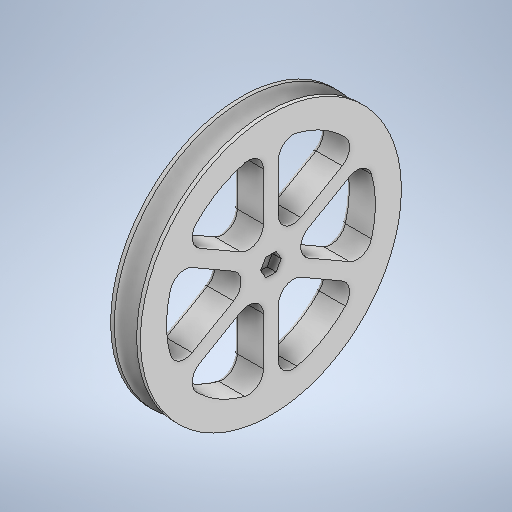
# Autodesk Inventor part: PLA Wheel Frame
Saved by Autodesk Inventor 2025.2 (Build 292293000, 293)
## iProperties
Created: 2025-01-16
Part Number: PLA Wheel Frame
Material: Generic
Document SubType Name: Modeling
Designer: Matt Tidd
Density: 1 g/cm^3
Appearance: Default
Author: Matt Tidd
Autodesk Inventor part; units mm, degrees
ref_plane "YZ Plane" through (0, 0, 0) normal (1, 0, 0) x (0, 1, 0)
ref_plane "XZ Plane" through (0, 0, 0) normal (0, 1, 0) x (-1, 0, 0)
ref_plane "XY Plane" through (0, 0, 0) normal (0, 0, 1) x (1, 0, 0)
sketch "Sketch1" plane through (0, 0, 0) normal (1, 0, 0) x (0, 1, 0)
  circle A0 centre (0, 0) radius 6
  line L0 (6, 3.4737) -> (6.0083, -3.4593)
  line L1 (6.0083, -3.4593) -> (0.0083, -6.933)
  line L2 (0.0083, -6.933) -> (-6, -3.4737)
  line L3 (-6, -3.4737) -> (-6.0083, 3.4593)
  line L4 (-6.0083, 3.4593) -> (-0.0083, 6.933)
  line L5 (-0.0083, 6.933) -> (6, 3.4737)
  circle A1 centre (0, 0) radius 20
  dimension "d0" = 12
  dimension "d1" = 40
  constraints: 12 end point, 3 coincident, 2 centre point, 13 other
  measures "d0" diameter of A0
  measures "d1" diameter of A1
extrude "Extrusion1" add sketch "Sketch1" along normal blind 20 contours A0 | L0 L1 L2 L3 L4 L5 | A1
sketch "Sketch2" plane through (20, 0, 0) normal (1, 0, 0) x (0, 0, -1)
  circle A0 centre (0, 0) radius 6
  line L0 (-6.934, 0) -> (-3.467, 6.005)
  line L1 (-3.467, 6.005) -> (3.467, 6.005)
  line L2 (3.467, 6.005) -> (6.934, 0)
  line L3 (6.934, 0) -> (3.467, -6.005)
  line L4 (3.467, -6.005) -> (-3.467, -6.005)
  line L5 (-3.467, -6.005) -> (-6.934, 0)
  point P0 (0, 6)
  dimension "d4" = 12
  constraints: 12 end point, 2 coincident, 1 vertical alignment, 15 other
extrude "Extrusion2" cut sketch "Sketch2" against normal blind 6 contours A0 | L0 L1 L2 L3 L4 L5
sketch "Sketch3" plane through (0, 0, 0) normal (-1, 0, 0) x (0, 0, 1)
  circle A0 centre (0, 0) radius 15
  dimension "d7" = 30
  constraints: 1 centre point, 1 coincident
  measures "d7" diameter of A0
extrude "Extrusion3" cut sketch "Sketch3" against normal blind 6
sketch "Sketch4" plane through (6, 0, 0) normal (-1, 0, 0) x (0, 0, 1)
  circle A0 centre (0, 0) radius 6
  dimension "d10" = 12
  constraints: 1 centre point, 1 coincident
  measures "d10" diameter of A0
extrude "Extrusion4" cut sketch "Sketch4" against normal blind 2
sketch "Sketch5" plane through (8, 0, 0) normal (-1, 0, 0) x (0, 0, 1)
  circle A0 centre (0, 0) radius 1.5
  dimension "d13" = 3
  constraints: 1 centre point, 1 coincident
  measures "d13" diameter of A0
extrude "Extrusion5" cut sketch "Sketch5" against normal through all
sketch "Sketch6" plane through (0, 0, 0) normal (-1, 0, 0) x (0, 0, 1)
  circle A0 centre (0, 0) radius 20 projected
  point P0 (0, 20)
  constraints: 1 vertical alignment, 1 other
ref_plane "Work Plane1" through (0, 20, 0) normal (0, 1, 0) x (-1, 0, 0)
sketch "Sketch7" plane through (0, 20, 0) normal (0, 1, 0) x (-1, 0, 0)
  line L0 (0, 0) -> (-20, 0) construction
  line L1 (-20, -3.467) -> (-20, 3.467) construction
  line L2 (-20, 5) -> (-20, -5) construction
  line L3 (-20, -3.467) -> (-20, -6.934) construction
  line L4 (-20, -5) -> (0, -5) construction
  line L5 (-20, -5) -> (0, -5)
  line L6 (0, -5) -> (0, 5)
  line L7 (0, 5) -> (-20, 5)
  line L8 (-20, 5) -> (-20, -5)
  dimension "d22" = 10
  dimension "d23" = 20
  dimension "d24" = 90
  dimension "d25" = 20
  dimension "d26" = 10
  constraints: 14 end point, 2 parallel, 2 perpendicular, 1 horizontal, 1 midpoint, 1 point on line
  measures "d22" distance of L2.start L2.end
  measures "d23" distance of L2.end L4.end
  measures "d24" angle of L4 L2
  measures "d25" distance of L7.end L6.end
  measures "d26" distance of L6.end L5.end
extrude "Extrusion6" add sketch "Sketch7" along normal blind 50 and the other way blind 2
pattern_circular "Circular Pattern1" count 6 over 360 about axis through (8, 0, 0) along (1, 0, 0) of "Extrusion6"
fillet "Fillet1" radius 10 12 edges at (10, 19.3649, 5) (10, 19.3649, -5) (10, 14.0126, -14.2705) (10, 5.3523, -19.2705) (10, -5.3523, -19.2705) (10, -14.0126, -14.2705) (10, -19.3649, -5) (10, -19.3649, 5) (10, -14.0126, 14.2705) (10, -5.3523, 19.2705) (10, 5.3523, 19.2705) (10, 14.0126, 14.2705)
sketch "Sketch9" plane through (0, 0, 0) normal (-1, 0, 0) x (0, 0, 1)
  circle A0 centre (0, 0) radius 1.5 projected
  circle A1 centre (0, 0) radius 70
  circle A2 centre (0, 0) radius 80
  circle A3 centre (0, 0) radius 87.5
  dimension "d37" = 160
  dimension "d42" = 175
  constraints: 3 centre point, 3 coincident
  measures "d37" diameter of A2
  measures "d42" diameter of A3
extrude "Extrusion7" add sketch "Sketch9" against normal up to surface (20 mm away) contours A2 | A3
fillet "Fillet2" radius 10 12 edges at (10, -69.8212, 5) (10, -69.8212, -5) (10, -39.2407, 57.9669) (10, -30.5805, 62.9669) (10, 30.5805, 62.9669) (10, 39.2407, 57.9669) (10, 69.8212, 5) (10, 69.8212, -5) (10, 39.2407, -57.9669) (10, 30.5805, -62.9669) (10, -30.5805, -62.9669) (10, -39.2407, -57.9669)
fillet "Fillet3" radius 2.5 48 edges at (0, -40.6873, -52.7199) (0, -25.349, -33.9057) (0, -20.9807, -6.3397) (0, -17.3205, -10) (0, -15.9807, -15) (0, -42.0377, -5) (0, -66.0004, -8.8763) (0, -60.6218, -35) (0, -16.6887, -38.9057) (0, -5, -21.3397) (0, 0, -20) (0, 5, -21.3397) (0, 16.6887, -38.9057) (0, 25.3131, -61.5962) (0, 0, -70) (0, -25.3131, -61.5962) (0, -15.9807, 15) (0, -17.3205, 10) (0, -20.9807, 6.3397) (0, -25.349, 33.9057) (0, -40.6873, 52.7199) (0, -60.6218, 35) (0, -66.0004, 8.8763) (0, -42.0377, 5) (0, 5, 21.3397) (0, 0, 20) (0, -5, 21.3397) (0, 16.6887, 38.9057) (0, 25.3131, 61.5962) (0, 0, 70) (0, -25.3131, 61.5962) (0, -16.6887, 38.9057) (0, 40.6873, -52.7199) (0, 60.6218, -35) (0, 66.0004, -8.8763) (0, 42.0377, -5) (0, 15.9807, -15) (0, 17.3205, -10) (0, 20.9807, -6.3397) (0, 25.349, -33.9057) (0, 25.349, 33.9057) (0, 40.6873, 52.7199) (0, 60.6218, 35) (0, 66.0004, 8.8763) (0, 42.0377, 5) (0, 20.9807, 6.3397) (0, 17.3205, 10) (0, 15.9807, 15)
ref_plane "Work Plane2" through (0, 87.5, 0) normal (0, 1, 0) x (1, 0, 0)
sketch "Sketch11" plane through (0, 87.5, 0) normal (0, 1, 0) x (1, 0, 0)
  line L0 (0, 0) -> (20, 0) construction
  line L1 (20, -3.467) -> (20, 3.467) construction
  point P0 (10, 0)
  constraints: 2 end point, 2 midpoint
ref_plane "Work Plane3" through (10, 87.5, 0) normal (0, 0, 1) x (1, 0, 0)
sketch "Sketch12" plane through (10, 87.5, 0) normal (0, 0, 1) x (1, 0, 0)
  line L0 (-10, 0) -> (10, 0) projected
  line L1 (-7.5, 0) -> (7.5, 0)
  line L2 (7.5, 0) -> (7.5, -7.5)
  line L3 (7.5, -7.5) -> (-7.5, -7.5)
  line L4 (-7.5, -7.5) -> (-7.5, 0)
  point P0 (-10, -87.5)
  dimension "d49" = 15
  dimension "d50" = 7.5
  constraints: 8 end point, 2 parallel, 1 horizontal, 1 perpendicular, 1 point on line
  measures "d49" distance of L2.end L3.end
  measures "d50" distance of L1.end L2.end
sketch "Sketch13" plane through (6, 0, 0) normal (-1, 0, 0) x (0, 0, 1)
  point P0 (0, 0)
  point P1 (0, 0)
  constraints: 1 coincident
ref_plane "Work Plane4" through (6, 0, 0) normal (0, 1, 0) x (1, 0, 0)
sketch "Sketch14" plane through (6, 0, 0) normal (0, 1, 0) x (1, 0, 0)
  line L0 (-24.0792, 0) -> (31.5972, 0) construction
  point P0 (-6, 0)
  constraints: 2 end point, 1 horizontal
revolve "Revolution1" cut sketch "Sketch12" angle 360 about axis through (-18.0792, 0, 0) along (1, 0, 0)
fillet "Fillet5" radius 7.5 2 edges at (2.5, -80, 0) (17.5, -80, 0)
body "Solid1"
